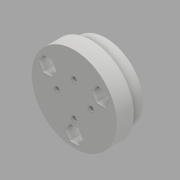
# Autodesk Inventor part: Arm - slew column A
Saved by Autodesk Inventor 2017 (Build 210142000, 142)
## iProperties
Created: 2017-06-05
Part Number: Arm - slew column A
Material: Generic
Document SubType Name: Modeling
Designer: Ali
Density: 1 g/cm^3
Appearance: Default
Author: Ali
Autodesk Inventor part; units mm, degrees
ref_plane "YZ Plane" through (0, 0, 0) normal (1, 0, 0) x (0, 1, 0)
ref_plane "XZ Plane" through (0, 0, 0) normal (0, 1, 0) x (-1, 0, 0)
ref_plane "XY Plane" through (0, 0, 0) normal (0, 0, 1) x (1, 0, 0)
sketch "Sketch1" plane through (0, 0, 0) normal (0, 1, 0) x (-1, 0, 0)
  circle A0 centre (0, 0) radius 8 construction
  circle A1 centre (8, 0) radius 1 construction
  circle A2 centre (0, -8) radius 1 construction
  circle A3 centre (-8, 0) radius 1 construction
  circle A4 centre (0, 8) radius 1 construction
  circle A5 centre (13, 0) radius 2 construction
  circle A6 centre (-6.5, 11.2583) radius 2 construction
  circle A7 centre (-6.5, -11.2583) radius 2 construction
  line L0 (13, 0) -> (0, 0)
  line L1 (0, 0) -> (0, -5.456)
  circle A8 centre (0, 0) radius 20
  dimension "d0" = 16
  dimension "d1" = 2
  dimension "d2" = 2
  dimension "d3" = 2
  dimension "d4" = 2
  dimension "d5" = 4
  dimension "d8" = 360
  dimension "d10" = 13
  dimension "d11" = 90
  dimension "d12" = 40
  constraints: 9 centre point, 4 end point, 4 point on circle, 1 coincident, 1 point on line, 1 vertical, 7 other
  measures "d0" diameter of A0
  measures "d1" diameter of A1
  measures "d2" diameter of A2
  measures "d3" diameter of A3
  measures "d4" diameter of A4
  measures "d5" diameter of A5
  measures "d10" distance of point (0, 0) L0.start
  measures "d11" angle of L0 L1
  measures "d12" diameter of A8
extrude "Extrusion1" add sketch "Sketch1" along normal blind 8
sketch "Sketch2" plane through (0, 8, 0) normal (0, 1, 0) x (1, 0, 0)
  circle A0 centre (0, 0) radius 17.5
  dimension "d15" = 35
  constraints: 1 centre point, 1 coincident
  measures "d15" diameter of A0
extrude "Extrusion2" add sketch "Sketch2" along normal blind 6.8
sketch "Sketch3" plane through (0, 14.8, 0) normal (0, 1, 0) x (1, 0, 0)
  circle A0 centre (0, -8) radius 1 construction
  circle A1 centre (-8, 0) radius 1 construction
  circle A2 centre (0, 8) radius 1 construction
  circle A3 centre (8, 0) radius 1 construction
  point P0 (0, 0)
hole "Hole1" at (0, 14.8, -8) at (-8, 14.8, 0) at (0, 14.8, 8) at (8, 14.8, 0) direction (0, -1, 0) diameter 2.3 end through all counterbore diameter 5.5 counterbore depth 6
sketch "Sketch4" plane through (0, 14.8, 0) normal (0, 1, 0) x (1, 0, 0)
  circle A0 centre (0, 0) radius 14.5
  point P0 (0, 14.5)
  point P1 (-12.5574, -7.25)
  point P2 (12.5574, -7.25)
  dimension "d27" = 29
  dimension "d30" = 360
  constraints: 1 coincident, 1 vertical alignment, 6 other
hole "Hole2" at (0, 14.8, -14.5) at (-12.5574, 14.8, 7.25) at (12.5574, 14.8, 7.25) direction (0, -1, 0) diameter 4.3 end through all
sketch "Sketch5" plane through (0, 0, 0) normal (0, -1, 0) x (1, 0, 0)
  circle A0 centre (-12.5574, 7.25) radius 2.15 construction
  circle A1 centre (12.5574, 7.25) radius 2.15 construction
  circle A2 centre (0, -14.5) radius 2.15 construction
  line L0 (4.0415, -14.5) -> (2.0207, -18)
  line L1 (2.0207, -18) -> (-2.0207, -18)
  line L2 (-2.0207, -18) -> (-4.0415, -14.5)
  line L3 (-4.0415, -14.5) -> (-2.0207, -11)
  line L4 (-2.0207, -11) -> (2.0207, -11)
  line L5 (2.0207, -11) -> (4.0415, -14.5)
  line L6 (14.5781, 10.75) -> (16.5988, 7.25)
  line L7 (10.5366, 10.75) -> (14.5781, 10.75)
  line L8 (8.5159, 7.25) -> (10.5366, 10.75)
  line L9 (10.5366, 3.75) -> (8.5159, 7.25)
  line L10 (14.5781, 3.75) -> (10.5366, 3.75)
  line L11 (16.5988, 7.25) -> (14.5781, 3.75)
  line L12 (-16.5988, 7.25) -> (-14.5781, 10.75)
  line L13 (-14.5781, 3.75) -> (-16.5988, 7.25)
  line L14 (-10.5366, 3.75) -> (-14.5781, 3.75)
  line L15 (-8.5159, 7.25) -> (-10.5366, 3.75)
  line L16 (-10.5366, 10.75) -> (-8.5159, 7.25)
  line L17 (-14.5781, 10.75) -> (-10.5366, 10.75)
  point P0 (0, 0)
  dimension "d39" = 7
  dimension "d42" = 360
  constraints: 36 end point, 1 coincident, 50 other
  measures "d39" distance between parallel lines of L5 L2
extrude "Extrusion3" cut sketch "Sketch5" against normal blind 6
body "Solid1"
